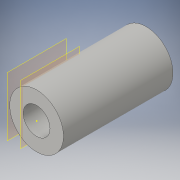
# Autodesk Inventor part: Threaded Rod Coupler
Saved by Autodesk Inventor 2016 (Build 200138000, 138)
## iProperties
Created: 2016-04-14
Part Number: Threaded Rod Coupler
Material: Generic
Document SubType Name: Modeling
Designer: rmarkowi
Density: 1 g/cm^3
Appearance: Default
Author: rmarkowi
Autodesk Inventor part; units mm, degrees
ref_plane "XZ Plane" through (0, 0, 0) normal (0, 1, 0) x (-1, 0, 0)
ref_plane "XY Plane" through (0, 0, 0) normal (0, 0, 1) x (1, 0, 0)
sketch "Sketch1" plane through (0, 0, 0) normal (0, 0, 1) x (1, 0, 0)
  circle A0 centre (0, 0) radius 12.7
  circle A1 centre (0, 0) radius 6.35
  dimension "d0" = 25.4
  dimension "d1" = 12.7
  constraints: 2 centre point, 2 coincident
  measures "d0" diameter of A0
  measures "d1" diameter of A1
extrude "Extrusion1" add sketch "Sketch1" against normal blind 25.4
sketch "Sketch2" plane through (0, 0, 0) normal (0, 1, 0) x (-1, 0, 0)
  point P0 (0, 0)
ref_plane "Work Plane2" through (-12.7, 0, 0) normal (1, 0, 0) x (0, 1, 0)
ref_plane "Work Plane1" through (-6.35, 0, 0) normal (1, 0, 0) x (0, 1, 0)
sketch "Sketch3" plane through (-6.35, 0, 0) normal (1, 0, 0) x (0, 1, 0)
  line L0 (-12.7, -25.4) -> (12.7, -25.4) construction
  line L1 (0, -25.4) -> (0, 0) construction
  circle A0 centre (0, -12.7) radius 2.55
  dimension "d6" = 5.1
  constraints: 2 end point, 2 midpoint, 1 centre point, 1 vertical
  measures "d6" diameter of A0
sketch "Sketch4" plane through (-12.7, 0, 0) normal (1, 0, 0) x (0, 1, 0)
  line L0 (-12.7, -25.4) -> (12.7, -25.4) construction
  line L1 (0, -25.4) -> (0, 0) construction
  circle A0 centre (0, -12.7) radius 2.65
  dimension "d7" = 5.3
  constraints: 2 end point, 2 midpoint, 1 centre point, 1 vertical
  measures "d7" diameter of A0
loft "Loft1" cut profiles "Sketch3", "Sketch4"
sketch "Sketch5" plane through (0, 0, -25.4) normal (0, 0, -1) x (-1, 0, 0)
  circle A0 centre (0, 0) radius 6.35 projected
  circle A1 centre (0, 0) radius 12.7
  constraints: 1 centre point, 1 coincident
extrude "Extrusion2" add sketch "Sketch5" along normal blind 6.35 contours A0 | A1
sketch "Sketch6" plane through (0, 0, -31.75) normal (0, 0, -1) x (-1, 0, 0)
  circle A0 centre (0, 0) radius 12.7
  circle A1 centre (0, 0) radius 3.175
  dimension "d14" = 6.35
  constraints: 2 centre point, 2 coincident
  measures "d14" diameter of A1
extrude "Extrusion3" add sketch "Sketch6" along normal blind 20
sketch "Sketch7" plane through (-6.35, 0, 0) normal (1, 0, 0) x (0, 1, 0)
  line L0 (-12.7, -51.75) -> (12.7, -51.75) construction
  line L1 (0, -51.75) -> (0, -31.75) construction
  line L2 (-3.175, -31.75) -> (3.175, -31.75) construction
  circle A0 centre (0, -41.75) radius 2.55
  point P0 (0, 0)
  dimension "d17" = 5.1
  constraints: 3 midpoint, 2 end point, 1 centre point
  measures "d17" diameter of A0
sketch "Sketch8" plane through (-12.7, 0, 0) normal (1, 0, 0) x (0, 1, 0)
  line L0 (-12.7, -51.75) -> (12.7, -51.75) construction
  line L1 (0, -51.75) -> (0, -31.75) construction
  line L2 (-3.175, -31.75) -> (3.175, -31.75) construction
  circle A0 centre (0, -41.75) radius 2.65
  point P0 (0, 0)
  dimension "d18" = 5.3
  constraints: 3 midpoint, 2 end point, 1 centre point
  measures "d18" diameter of A0
loft "Loft2" cut profiles "Sketch7", "Sketch8"
body "Solid1"
